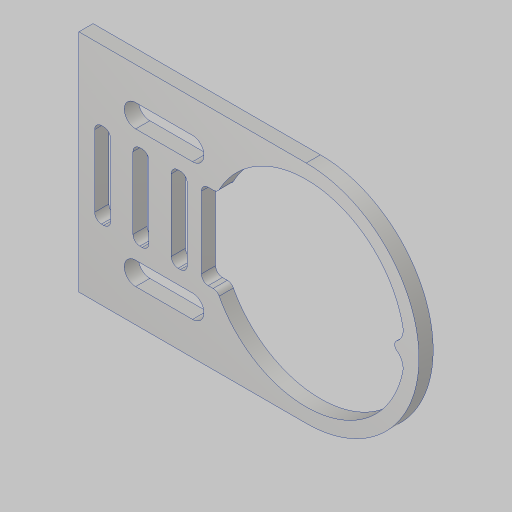
# Autodesk Inventor part: EL2-009
Saved by Autodesk Inventor 2023.5 (Build 275446000, 446)
## iProperties
Created: 2025-01-12
Part Number: EL2-009
Material: Aluminum 6061
Document SubType Name: Modeling
Designer: mavericks
Density: 2.7 g/cm^3
Appearance: Aluminum - Flat
Author: mavericks
Autodesk Inventor part; units mm, degrees
ref_plane "YZ Plane" through (0, 0, 0) normal (1, 0, 0) x (0, 1, 0)
ref_plane "XZ Plane" through (0, 0, 0) normal (0, 1, 0) x (-1, 0, 0)
ref_plane "XY Plane" through (0, 0, 0) normal (0, 0, 1) x (1, 0, 0)
sketch "Sketch1" plane through (0, 0, 0) normal (0, 0, 1) x (1, 0, 0)
  line L0 (0, 0) -> (50.8, 0) construction
  line L1 (50.8, 0) -> (50.8, 50.3682) construction
  line L2 (50.8, 50.3682) -> (0, 50.3682) construction
  line L3 (0, 50.3682) -> (0, 0) construction
  circle A0 centre (50.8, 25.1841) radius 25.1841 construction
  line L4 (0, 0) -> (50.8, 0)
  line L5 (50.8, 0) -> (50.8, 50.3682) construction
  line L6 (50.8, 50.3682) -> (0, 50.3682)
  line L7 (0, 50.3682) -> (0, 0)
  arc A1 (50.8, 0) -> (50.8, 50.3682) centre (50.8, 25.1841) ccw
  dimension "d0" = 50.8
  dimension "d1" = 50.3682
  constraints: 16 end point, 4 parallel, 2 horizontal, 2 perpendicular, 2 point on circle, 1 centre point, 1 coincident, 1 midpoint, 1 vertical alignment, 2 other
  measures "d0" distance of L2.end L1.end
  measures "d1" distance of L0.end L1.end
extrude "Extrusion1" add sketch "Sketch1" along normal blind 3.175
sketch "Sketch2" plane through (0, 0, 3.175) normal (0, 0, 1) x (1, 0, 0)
  arc A0 (50.8, 0) -> (50.8, 50.3682) centre (50.8, 25.1841) ccw projected
  arc A1 (57.1075, 4.0982) -> (50.8, 47.1932) centre (50.8, 25.1841) ccw
  line L0 (27.3812, 15.6959) -> (33.7312, 15.6959)
  line L1 (33.7312, 15.6959) -> (33.7312, 34.7459)
  line L2 (33.7312, 34.7459) -> (27.3812, 34.7459)
  line L3 (27.3812, 34.7459) -> (27.3812, 15.6959)
  line L4 (27.3812, 15.6959) -> (33.7312, 34.7459) construction
  line L5 (33.7312, 15.6959) -> (27.3812, 34.7459) construction
  arc A2 (50.8, 47.1932) -> (30.9765, 34.7459) centre (50.8, 25.1841) ccw
  arc A3 (30.9411, 15.6959) -> (57.1075, 4.0982) centre (50.8, 25.1841) ccw
  line L6 (0, 50.3682) -> (0, 0) projected
  line L7 (50.8, 50.3682) -> (0, 50.3682) projected
  point P0 (30.5562, 25.2209)
  dimension "d6" = 3.175
  dimension "d7" = 6.35
  dimension "d8" = 19.05
  dimension "d9" = 12.4473
  dimension "d10" = 27.3812
  dimension "d11" = 15.6223
  constraints: 12 end point, 7 point on circle, 3 centre point, 2 coincident, 2 midpoint, 2 parallel, 2 point on line, 1 horizontal, 1 perpendicular
  measures "d6" radial gap between concentric circles of A0 A1
  measures "d7" distance of L2.end L1.end
  measures "d8" distance of L0.end L1.end
  measures "d9" vertical distance of A1.end L1.end
  measures "d10" distance between parallel lines of L3 L6
  measures "d11" distance between parallel lines of L7 L2
extrude "Extrusion2" cut sketch "Sketch2" against normal blind 3.175
sketch "Sketch3" plane through (0, 0, 3.175) normal (0, 0, 1) x (1, 0, 0)
  circle A0 centre (71.755, 25.1433) radius 1.1913
  line L0 (30.9411, 15.6959) -> (27.3812, 15.6959) projected
  line L1 (27.3812, 15.6959) -> (27.3812, 34.7459) projected
  line L2 (27.3812, 34.7459) -> (30.9765, 34.7459) projected
  arc A1 (30.9411, 15.6959) -> (30.9765, 34.7459) centre (50.8, 25.1841) ccw projected
  arc A2 (50.8, 0) -> (50.8, 50.3682) centre (50.8, 25.1841) ccw projected
  line L3 (50.8, 50.3682) -> (0, 50.3682) projected
  line L4 (0, 50.3682) -> (0, 0) projected
  line L5 (0, 0) -> (50.8, 0) projected
  point P0 (72.8091, 25.1433)
  point P1 (72.8006, 24.5725)
  point P2 (72.8028, 25.71)
  dimension "d14" = 2.3825
  dimension "d15" = 20.955
  constraints: 1 centre point, 1 horizontal alignment, 1 point on circle
  measures "d14" diameter of A0
  measures "d15" distance of A0.centre A1.centre
extrude "Extrusion3" add sketch "Sketch3" against normal up to surface (3.175 mm away) contours A1 A0 picked at (72.0601, 25.1427)
fillet "Fillet1" radius 3.302 2 edges at (72.8006, 24.5725, 1.5875) (72.8028, 25.71, 1.5875)
sketch "Sketch4" plane through (0, 0, 3.175) normal (0, 0, 1) x (1, 0, 0)
  line L0 (24.2062, 34.7459) -> (20.6502, 34.7459)
  line L1 (20.6502, 34.7459) -> (20.6502, 15.6959)
  line L2 (20.6502, 15.6959) -> (24.2062, 15.6959)
  line L3 (24.2062, 15.6959) -> (24.2062, 34.7459)
  line L4 (24.2062, 34.7459) -> (20.6502, 15.6959) construction
  line L5 (20.6502, 34.7459) -> (24.2062, 15.6959) construction
  line L6 (15.6502, 34.7459) -> (12.0942, 34.7459)
  line L7 (12.0942, 34.7459) -> (12.0942, 15.6959)
  line L8 (12.0942, 15.6959) -> (15.6502, 15.6959)
  line L9 (15.6502, 15.6959) -> (15.6502, 34.7459)
  line L10 (15.6502, 34.7459) -> (12.0942, 15.6959) construction
  line L11 (12.0942, 34.7459) -> (15.6502, 15.6959) construction
  line L12 (7.0942, 34.7459) -> (3.5382, 34.7459)
  line L13 (3.5382, 34.7459) -> (3.5382, 15.6959)
  line L14 (3.5382, 15.6959) -> (7.0942, 15.6959)
  line L15 (7.0942, 15.6959) -> (7.0942, 34.7459)
  line L16 (7.0942, 34.7459) -> (3.5382, 15.6959) construction
  line L17 (3.5382, 34.7459) -> (7.0942, 15.6959) construction
  line L18 (27.3812, 15.6959) -> (27.3812, 34.7459) projected
  line L19 (0, 50.3682) -> (0, 0) projected
  line L20 (27.3812, 34.7459) -> (30.9765, 34.7459) projected
  line L21 (27.9527, 9.9682) -> (10.1473, 9.9682) construction
  line L22 (25.4, 12.5209) -> (12.7, 12.5209)
  line L23 (12.7, 7.4155) -> (25.4, 7.4155)
  arc A0 (25.4, 7.4155) -> (25.4, 12.5209) centre (25.4, 9.9682) ccw
  arc A1 (12.7, 12.5209) -> (12.7, 7.4155) centre (12.7, 9.9682) ccw
  line L24 (27.9527, 40.4736) -> (10.1473, 40.4736) construction
  line L25 (25.4, 43.0263) -> (12.7, 43.0263)
  line L26 (12.7, 37.9209) -> (25.4, 37.9209)
  arc A2 (25.4, 37.9209) -> (25.4, 43.0263) centre (25.4, 40.4736) ccw
  arc A3 (12.7, 43.0263) -> (12.7, 37.9209) centre (12.7, 40.4736) ccw
  line L27 (30.9411, 15.6959) -> (27.3812, 15.6959) projected
  point P0 (22.4282, 25.2209)
  point P1 (13.8722, 25.2209)
  point P2 (5.3162, 25.2209)
  point P3 (27.3812, 25.2209)
  point P4 (19.05, 9.9682)
  point P5 (19.05, 40.4736)
  point P6 (27.9527, 40.4736)
  point P7 (12.0942, 25.2209)
  dimension "d19" = 3.175
  dimension "d20" = 5
  dimension "d21" = 5
  dimension "d22" = 3.556
  dimension "d23" = 3.556
  dimension "d24" = 3.556
  dimension "d25" = 19.05
  dimension "d26" = 19.05
  dimension "d27" = 19.05
  dimension "d28" = 3.5382
  dimension "d29" = 5.1054
  dimension "d30" = 5.1054
  dimension "d33" = 12.7
  dimension "d34" = 12.7
  dimension "d35" = 3.175
  dimension "d36" = 3.175
  dimension "d37" = 19.05
  constraints: 52 end point, 13 point on circle, 10 midpoint, 8 parallel, 8 tangent, 5 horizontal, 4 centre point, 4 point on line, 3 horizontal alignment, 3 perpendicular, 1 vertical alignment
  measures "d19" distance between parallel lines of L18 L3
  measures "d20" distance between parallel lines of L9 L1
  measures "d21" distance between parallel lines of L15 L7
  measures "d22" distance of L7.end L8.end
  measures "d23" distance of L1.end L2.end
  measures "d24" distance of L13.end L14.end
  measures "d25" distance of L14.end L12.start
  measures "d26" distance of L8.end L6.start
  measures "d27" distance of L2.end L0.start
  measures "d28" distance between parallel lines of L19 L13
  measures "d29" diameter of A1
  measures "d30" diameter of A3
  measures "d33" distance of A3.centre A2.centre
  measures "d34" distance of A1.centre A0.centre
  measures "d35" distance between parallel lines of L20 L26
  measures "d36" distance between parallel lines of L27 L22
  measures "d37" distance from line of L19 point (19.05, 9.968)
extrude "Extrusion4" cut sketch "Sketch4" against normal blind 25.4
fillet "Fillet2" radius 1.524 16 edges at (3.5382, 34.7459, 1.5875) (7.0942, 34.7459, 1.5875) (3.5382, 15.6959, 1.5875) (7.0942, 15.6959, 1.5875) (12.0942, 34.7459, 1.5875) (15.6502, 34.7459, 1.5875) (15.6502, 15.6959, 1.5875) (12.0942, 15.6959, 1.5875) (24.2062, 34.7459, 1.5875) (20.6502, 34.7459, 1.5875) (20.6502, 15.6959, 1.5875) (24.2062, 15.6959, 1.5875) (27.3812, 34.7459, 1.5875) (27.3812, 15.6959, 1.5875) (30.9411, 15.6959, 1.5875) (30.9765, 34.7459, 1.5875)
equation "\"d22\" = d23"
equation "\"d24\" = d23"
equation "\"d26\" = d25"
equation "\"d27\" = d25"
equation "\"d34\" = d33"
equation "\"d36\" = d35"
body "Solid1"
